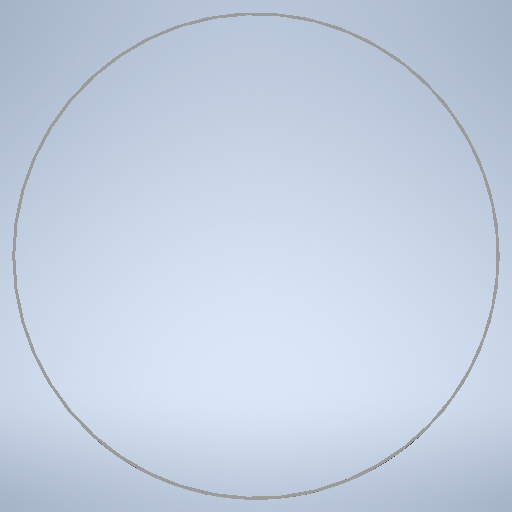
# Autodesk Inventor part: PNS-701 main shell D1200
Saved by Autodesk Inventor 2025.1 (Build 291241020, 241B)
## iProperties
Created: 2025-02-11
Part Number: PNS-701 main shell D1200
Material: Steel
Document SubType Name: Sheet Metal
Designer: pokla
Density: 7.85 g/cm^3
Flat Pattern Width: 190 cm
Flat Pattern Length: 303.167 cm
Flat Pattern Area: 57601.8 cm^2
Sheet Metal Rule: Default_mm
Sheet Metal Width: 1900.000 mm
Sheet Metal Length: 3031.674 mm
Sheet Metal Area: 5760180.963 mm^2
Appearance: Default
Mass: 309189 g
Surface Area: 132135 cm^2
Volume: 39387.1 cm^3
Flat Pattern Length: 296.886 cm
Flat Pattern Area: 56408.3 cm^2
Sheet Metal Width: 1900,000 mm
Sheet Metal Length: 2968,860 mm
Sheet Metal Area: 5640833,603 mm^2
Author: pokla
Sheet Metal Length: 2968.860 mm
Sheet Metal Area: 5640833.603 mm^2
Autodesk Inventor part; units mm, degrees
ref_plane "YZ Plane" through (0, 0, 0) normal (1, 0, 0) x (0, 1, 0)
ref_plane "XZ Plane" through (0, 0, 0) normal (0, 1, 0) x (-1, 0, 0)
ref_plane "XY Plane" through (0, 0, 0) normal (0, 0, 1) x (1, 0, 0)
sketch "Sketch1" plane through (0, 0, 0) normal (0, 1, 0) x (-1, 0, 0)
  line L0 (486, 1900) -> (480, 1900)
  line L1 (480, 1900) -> (480, 0)
  line L2 (480, 0) -> (486, 0)
  line L3 (486, 0) -> (486, 1900)
  line L4 (0, 0) -> (0, 1673.0415)
  point P0 (483, 0)
  dimension "d0" = 6
  dimension "d1" = 1900
  dimension "d2" = 960
  constraints: 10 end point, 2 parallel, 1 coincident, 1 horizontal, 1 horizontal alignment, 1 midpoint, 1 perpendicular, 1 vertical
  measures "d0" distance between parallel lines of L1 L3
  measures "d1" distance of L2.end L0.start
  measures "d2" diameter of L1 L4
revolve "Revolution1" add sketch "Sketch1" angle 359.9 about axis through (0, 0, 0) along (0, 0, 1)
sketch "Sketch2" plane through (0, 0, 0) normal (0, 1, 0) x (-1, 0, 0)
  circle A0 centre (0, 400) radius 265
  line L0 (480, 1900) -> (-480, 1900) projected
  line L1 (110, 1700) -> (-110, 1700) construction
  line L2 (110, 1790) -> (-110, 1790)
  line L3 (-110, 1610) -> (110, 1610)
  arc A1 (110, 1610) -> (110, 1790) centre (110, 1700) ccw
  arc A2 (-110, 1790) -> (-110, 1610) centre (-110, 1700) ccw
  line L4 (200, 1700) -> (-200, 1700) construction
  point P0 (0, 0)
  point P1 (479.9993, 1900)
  point P2 (0, 1700)
  dimension "d4" = 530
  dimension "d12" = 400
  dimension "d15" = 200
  dimension "d16" = 400
  dimension "d17" = 180
  constraints: 10 end point, 6 point on circle, 4 tangent, 3 centre point, 2 vertical alignment, 1 horizontal, 1 midpoint, 1 parallel
  measures "d4" diameter of A0
  measures "d12" distance of A0.centre point (0, 0)
  measures "d15" distance between parallel lines of L1 L0
  measures "d16" distance of L4.start L4.end
  measures "d17" distance between parallel lines of L3 L2
extrude "Extrusion1" cut sketch "Sketch2" against normal through all contours A0
sketch "floor angle sketch" plane through (0, 0, 0) normal (0, 0, 1) x (1, 0, 0)
  line L0 (0, 0) -> (0, -267.717)
  line L1 (0, -267.717) -> (0, 0)
  line L2 (0, 0) -> (72.6903, -155.8849)
  line L3 (0, 0) -> (-51.6219, -73.7237)
  line L4 (0, 0) -> (51.6219, -73.7237)
  dimension "Feeder_way_angle" = 335
  dimension "Feeder_way_line" = 172
  dimension "Outer_way_line" = 90
  dimension "Inner_way_line" = 90
  dimension "Outer_way_angle" = 325
  dimension "Inner_way_angle" = 35
  constraints: 10 end point, 1 collinear, 1 vertical
  measures "Feeder_way_line" distance of L0.start L2.end
  measures "Outer_way_line" distance of L0.start L4.end
  measures "Inner_way_line" distance of L0.start L3.end
  measures "Inner_way_angle" angle of L0 L3
ref_plane "Feeder Plane" through (0, 0, -10) normal (0.9063078, 0.4226183, 0) x (0, 0, 1)
sketch "Feeder horisont hight angle" plane through (0, 0, -10) normal (0.9063078, 0.4226183, 0) x (0, 0, 1)
  line L0 (1910, -480) -> (1910, 480) construction
  line L1 (10, 0) -> (1910, 0) construction
  line L2 (1229.4078, 0) -> (1510, 486)
  line L3 (10, 486) -> (1910, 486) construction
  line L4 (1510, 486) -> (1510, 0) construction
  point P0 (1910, -202.8568)
  point P1 (1910, -203.6157)
  dimension "d34" = 1500
  dimension "d35" = 30
  constraints: 6 end point, 3 point on line, 1 midpoint, 1 perpendicular
  measures "d34" distance of L3.start L2.end
  measures "d35" angle of L2 L4
ref_plane "Feeder Work Plane" through (0, 0, 1219.4078) normal (0.3659982, -0.7848856, 0.5) x (0.9063078, 0.4226183, 0)
sketch "Sketch8" plane through (0, 0, 1219.4078) normal (0.3659982, -0.7848856, 0.5) x (0.9063078, 0.4226183, 0)
  circle A0 centre (0, 0) radius 86
  point P0 (0, -1056.0381)
  point P1 (0, 0)
  point P2 (0, 0)
  point P3 (0, 0)
  dimension "d36" = 172
  constraints: 1 centre point, 1 coincident, 1 vertical alignment
  measures "d36" diameter of A0
extrude "Feeder Extrusion" cut sketch "Sketch8" along normal through all
ref_plane "Inner Plane" through (0, 0, 0) normal (-0.819152, 0.5735764, 0) x (-0.5735764, -0.819152, 0)
sketch "Inner horisont hight angle" plane through (0, 0, 0) normal (-0.819152, 0.5735764, 0) x (-0.5735764, -0.819152, 0)
  line L0 (486, 1900) -> (-486, 1900) construction
  line L1 (486, 0) -> (486, 1900) construction
  line L2 (0, 0) -> (0, 1900) construction
  line L3 (0, 1300) -> (486, 1300) construction
  line L4 (486, 1300) -> (0, 1300)
  point P0 (278.7581, 1900)
  point P1 (278.0629, 1900)
  dimension "d40" = 0
  dimension "d41" = 1300
  constraints: 6 end point, 3 point on line, 1 midpoint, 1 perpendicular
  measures "d40" distance between parallel lines of L4 L3
  measures "d41" distance of L1.start L3.end
ref_plane "Inner Work Plane" through (0, 0, 1300) normal (0.5735764, 0.819152, 0) x (-0.819152, 0.5735764, 0)
sketch "Sketch10" plane through (0, 0, 1300) normal (0.5735764, 0.819152, 0) x (-0.819152, 0.5735764, 0)
  circle A0 centre (0, 0) radius 45.5
  point P0 (0, -1300)
  point P1 (0, 0)
  point P2 (0, 0)
  point P3 (0, 0)
  dimension "d42" = 91
  constraints: 1 centre point, 1 coincident
  measures "d42" diameter of A0
extrude "Inner Extrusion" cut sketch "Sketch10" against normal through all
ref_plane "Outer Plane" through (0, 0, 0) normal (-0.819152, -0.5735764, 0) x (0.5735764, -0.819152, 0)
sketch "Sketch11" plane through (0, 0, 0) normal (-0.819152, -0.5735764, 0) x (0.5735764, -0.819152, 0)
  line L0 (0, 0) -> (0, 1900)
  line L1 (486, 1900) -> (-486, 1900) projected
  line L2 (0, 700) -> (486, 700)
  line L3 (486, 0) -> (486, 1900) projected
  line L4 (486, 700) -> (0, 700)
  point P0 (-278.7581, 1900)
  point P1 (-279.4526, 1900)
  dimension "d45" = 0
  dimension "d46" = 700
  constraints: 6 end point, 3 point on line, 1 midpoint, 1 perpendicular
  measures "d45" distance between parallel lines of L4 L2
  measures "d46" distance of L3.start L2.end
ref_plane "Work Plane9" through (0, 0, 700) normal (-0.5735764, 0.819152, 0) x (-0.819152, -0.5735764, 0)
sketch "Sketch12" plane through (0, 0, 700) normal (-0.5735764, 0.819152, 0) x (-0.819152, -0.5735764, 0)
  circle A0 centre (0, 0) radius 46
  point P0 (0, -700)
  point P1 (0, 0)
  point P2 (0, 0)
  point P3 (0, 0)
  dimension "d47" = 92
  constraints: 1 centre point, 1 coincident
  measures "d47" diameter of A0
extrude "Extrusion6" cut sketch "Sketch12" against normal through all
equation "\"d2\" = MAIN_filter_diam"
equation "\"d4\" = Accsess_hatch_diameter"
equation "\"d16\" = Charging_hatch_width"
equation "\"d17\" = Charging_hatch_hight"
equation "\"d34\" = Feedr_hight"
equation "\"d35\" = Feeder_horisont_hight_angle"
equation "\"BendRadius\" = Thickness"
equation "\"BendReliefWidth\" = Thickness"
equation "\"BendReliefDepth\" = 0.5 * Thickness"
equation "\"CornerReliefSize\" = 4 * Thickness"
equation "\"MinimumRemnant\" = 2 * Thickness"
equation "\"TransitionRadius\" = BendRadius"
equation "\"JacobiRadiusSize\" = BendRadius"
equation "\"GapSize\" = Thickness"
equation "\"MAIN_filter_diam\" = 960"
equation "\"Accsess_hatch_diameter\" = 530"
equation "\"Disherd_head_hight\" = 253.28919"
equation "\"Charging_hatch_width\" = 400"
equation "\"Charging_hatch_hight\" = 180"
equation "\"Feeder_floor_angle\" = 60deg"
equation "\"Feedr_hight\" = 1500"
equation "\"Feeder_horisont_hight_angle\" = 30deg"
equation "\"Thickness\" = 6"
body "Solid1"
